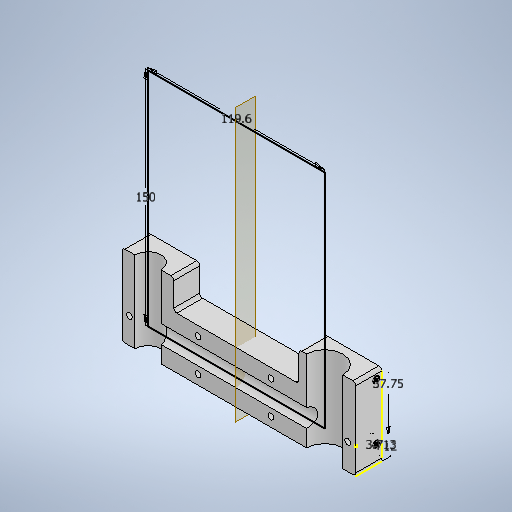
# Autodesk Inventor part: BottomBase
Saved by Autodesk Inventor 2026 (Build 300175050, 175E)
## iProperties
Created: 2025-12-10
Part Number: BottomBase
Material: Generic
Document SubType Name: Modeling
Designer: Nicholas M
Density: 1 g/cm^3
Appearance: Default
Author: Nicholas M
Autodesk Inventor part; units mm, degrees
ref_plane "YZ Plane" through (0, 0, 0) normal (1, 0, 0) x (0, 1, 0)
ref_plane "XZ Plane" through (0, 0, 0) normal (0, 1, 0) x (-1, 0, 0)
ref_plane "XY Plane" through (0, 0, 0) normal (0, 0, 1) x (1, 0, 0)
sketch "Sketch1" plane through (0, 0, 0) normal (0, 0, 1) x (1, 0, 0)
  line L0 (0, 0) -> (119.6, 0)
  line L1 (119.6, 0) -> (119.6, 150)
  line L2 (119.6, 150) -> (0, 150)
  line L3 (0, 150) -> (0, 0)
  dimension "d0" = 119.6
  dimension "d1" = 150
  constraints: 8 end point, 2 parallel, 1 horizontal, 1 perpendicular
  measures "d0" distance of L2.end L1.end
  measures "d1" distance of L1.end L0.end
sketch "Sketch2" plane through (0, 0, 0) normal (1, 0, 0) x (0, 1, 0)
  circle A0 centre (0, 0) radius 12.5
  circle A1 centre (0, 0) radius 6.125
  line L0 (-12.5, 0) -> (12.5, 0)
  line L1 (12.5, 0) -> (12.5, 12.5)
  line L2 (12.5, 12.5) -> (-12.5, 12.5)
  line L3 (-12.5, 12.5) -> (-12.5, 0)
  circle A2 centre (150, 0) radius 12.5
  circle A3 centre (150, 0) radius 6.125
  line L4 (137.5, 0) -> (162.5, 0)
  line L5 (162.5, 0) -> (162.5, 12.5)
  line L6 (162.5, 12.5) -> (137.5, 12.5)
  line L7 (137.5, 12.5) -> (137.5, 0)
  line L8 (-12.5, 12.5) -> (-17.5, 12.5)
  line L9 (-17.5, 12.5) -> (-17.5, 0)
  line L10 (-17.5, 0) -> (-12.5, 0)
  line L11 (-12.5, 0) -> (-12.5, 12.5)
  line L12 (12.5, 12.5) -> (17.5, 12.5)
  line L13 (17.5, 12.5) -> (17.5, 0)
  line L14 (17.5, 0) -> (12.5, 0)
  line L15 (12.5, 0) -> (12.5, 12.5)
  point P0 (6.125, 0)
  point P1 (-6.125, 0)
  point P2 (150, 0)
  point P3 (12.5, 0)
  dimension "d2" = 25
  dimension "d3" = 12.25
  dimension "d6" = 5
  dimension "d7" = 5
  dimension "d8" = 35
  constraints: 32 end point, 8 parallel, 6 horizontal, 4 coincident, 4 horizontal alignment, 4 perpendicular, 4 vertical, 2 centre point, 1 equal radius, 1 midpoint, 4 other
  measures "d3" diameter of A1
  measures "d6" distance between parallel lines of L9 L3
  measures "d7" distance of L13.end L14.end
  measures "d8" distance between parallel lines of L13 L9
extrude "Extrusion1" add sketch "Sketch2" along normal up to surface (119.6 mm away) contours L3 L2 A0 | A0 L0 A1 | L10 L9 L8 L3 | A0 L2 L1 | L1 L12 L13 L14 | A1 L0 picked at (10.2705, 0.9272) picked at (1.5282, 2.3311)
ref_plane "Work Plane1" through (59.8, 0, 0) normal (-1, 0, 0) x (0, 0, 1)
sketch "Sketch3" plane through (0, -17.5, 0) normal (0, -1, 0) x (1, 0, 0)
  line L0 (0, 12.5) -> (119.6, 12.5) projected
  line L1 (102.1, 12.5) -> (137.1, 12.5)
  line L2 (137.1, 12.5) -> (137.1, 0)
  line L3 (137.1, 0) -> (102.1, 0)
  line L4 (102.1, 0) -> (102.1, 12.5)
  line L5 (119.6, 12.5) -> (119.6, 0) projected
  circle A0 centre (119.6, 0) radius 8.925
  point P0 (0, 0)
  point P1 (119.6, 12.5)
  point P2 (128.525, 0)
  point P3 (110.675, 0)
  dimension "d9" = 35
  dimension "d33" = 17.85
  constraints: 8 end point, 2 parallel, 1 centre point, 1 coincident, 1 horizontal, 1 midpoint, 1 perpendicular, 1 point on line
  measures "d9" distance between parallel lines of L2 L4
  measures "d33" diameter of A0
extrude "Extrusion2" add sketch "Sketch3" against normal blind 55 contours L0 L5 A0 L3 L4 | L1 L2 L3 A0 L5 | A0 L3 L5 | L5 L3 A0
extrude "Extrusion4" cut sketch "Sketch3" along normal through all both and the other way through all contours A0 L3 L5 | L5 L3 A0
extrude "Extrusion3" cut sketch "Sketch2" along normal up to surface (119.6 mm away) contours A1 L0 picked at (1.5282, 2.3311)
mirror "Mirror1" about plane through (59.8, 0, 0) normal (-1, 0, 0) of "Extrusion2", "Extrusion4", "Extrusion3"
sketch "Sketch4" plane through (102.1, 17.5, 12.5) normal (0, 0, 1) x (1, 0, 0)
  line L0 (-119.6, -35) -> (35, -35) projected
  line L1 (0, 20) -> (35, 20) projected
  line L2 (0, 0) -> (0, 20) projected
  line L3 (-84.6, 0) -> (0, 0) projected
  line L4 (-84.6, 0) -> (-84.6, 20) projected
  line L5 (-84.6, 20) -> (-119.6, 20) projected
  line L6 (35, -35) -> (35, 20) projected
  line L7 (-119.6, -35) -> (-119.6, 20) projected
  point P0 (-102.1, -17.5)
extrude "Extrusion5" add sketch "Sketch4" along normal blind 5
sketch "Sketch5" plane through (102.1, 17.5, 0) normal (0, 0, -1) x (-1, 0, 0)
  circle A0 centre (16.425, -6.375) radius 2
  line L0 (-8.575, -11.375) -> (93.175, -11.375) projected
  line L1 (-8.575, 20) -> (-8.575, -11.375) projected
  circle A1 centre (65.675, -6.375) radius 2
  circle A2 centre (16.425, -28.625) radius 2
  circle A3 centre (65.675, -28.625) radius 2
  line L2 (93.175, -35) -> (93.175, -23.625) projected
  line L3 (93.175, -23.625) -> (-8.575, -23.625) projected
  circle A4 centre (-30, -17.5) radius 2
  circle A5 centre (117.6, -17.5) radius 2
  line L4 (-35, -35) -> (-35, 20) projected
  line L5 (119.6, -35) -> (119.6, 20) projected
  line L6 (16.425, -6.375) -> (16.425, -28.625) construction
  point P0 (102.1, -17.5)
  point P1 (16.425, -17.5)
  dimension "d18" = 4
  dimension "d19" = 5
  dimension "d20" = 25
  dimension "d23" = 49.25
  dimension "d26" = 22.25
  dimension "d29" = 27.5
  dimension "d30" = 5
  dimension "d38" = 5
  dimension "d39" = 2
  constraints: 6 centre point, 2 end point, 2 equal radius, 2 horizontal alignment, 2 vertical, 1 horizontal, 1 midpoint, 6 other
  measures "d18" diameter of A0
  measures "d19" distance from line of L0 L6.start
  measures "d20" distance from line of L1 L6.start
  measures "d23" distance of L6.start A1.centre
  measures "d26" distance of L6.start L6.end
  measures "d29" distance from line of L2 A3.centre
  measures "d30" distance from line of L3 A3.centre
  measures "d38" distance from line of L4 A4.centre
  measures "d39" distance from line of L5 A5.centre
extrude "Extrusion6" cut sketch "Sketch5" against normal blind 10
sketch "Sketch6" plane through (0, 37.5, 0) normal (0, 1, 0) x (1, 0, 0)
  circle A0 centre (0, 0) radius 12.325
  line L0 (-17.5, 0) -> (-17.5, -17.5) projected
  line L1 (-17.5, -17.5) -> (-21, -17.5)
  line L2 (-21, -17.5) -> (-21, 0)
  line L3 (-21, 0) -> (-17.5, 0)
  line L4 (-17.5, 0) -> (-17.5, -17.5)
  line L5 (-17.5, 0) -> (-8.925, 0) projected
  dimension "d34" = 24.65
  dimension "d40" = 3.5
  constraints: 8 end point, 2 parallel, 1 centre point, 1 coincident, 1 collinear, 1 horizontal, 1 perpendicular
  measures "d34" diameter of A0
  measures "d40" distance of L2.end L3.end
extrude "Extrusion7" cut sketch "Sketch6" against normal through all contours A0
extrude "Extrusion8" add sketch "Sketch6" against normal up to surface (55 mm away) contours L0 L1 L2 L3
fillet "Fillet1" radius 2 8 edges at (102.1, 17.5, 8.75) (17.5, 17.5, 8.75) (17.5, 37.5, 8.75) (102.1, 37.5, 8.75) (137.1, 37.5, 8.75) (137.1, -17.5, 8.75) (-21, 37.5, 8.75) (-21, -17.5, 8.75)
sketch "Sketch7" plane through (-21, -15.5, 17.5) normal (-1, 0, 0) x (0, 0, 1)
  circle A0 centre (-3.7125, 10) radius 2
  line L0 (0, 51) -> (0, 0) projected
  line L1 (-17.5, -2) -> (0, -2) projected
  circle A1 centre (-3.7125, 47.75) radius 2
  point P0 (-17.5, 15.5)
  dimension "d43" = 4
  dimension "d44" = 3.7125
  dimension "d45" = 12
  dimension "d49" = 37.75
  constraints: 2 centre point, 1 equal radius, 1 vertical alignment
  measures "d43" diameter of A0
  measures "d44" distance from line of L0 A0.centre
  measures "d45" distance from line of L1 A0.centre
  measures "d49" distance of A1.centre A0.centre
extrude "Extrusion9" cut sketch "Sketch7" against normal blind 5
extrude "Extrusion10" cut sketch "Sketch7" along normal blind 5 from surface at -158.1
equation "\"d7\" = d6"
equation "\"d9\" = d8"
body "Solid1"
